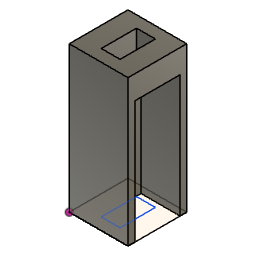
Sensor Lift (Autodesk Fusion 360 design; units mm, degrees)
Autodesk Fusion 360 part; units mm, degrees
note: some values were not read from the file. Set by a fixed rule: which sketch regions a step uses.
sketch "Sketch1" plane through (0, 0, 0) normal (0, 0, 1) x (1, 0, 0)
  line L0 (0, 0) -> (15, 0)
  line L1 (15, 0) -> (15, 15)
  line L2 (15, 15) -> (0, 15)
  line L3 (0, 15) -> (0, 0)
  line L4 (5.1406, 12.0446) -> (9.9406, 12.0446)
  line L5 (9.9406, 12.0446) -> (9.9406, 3.0446)
  line L6 (9.9406, 3.0446) -> (5.1406, 3.0446)
  line L7 (5.1406, 3.0446) -> (5.1406, 12.0446)
  dimension "d1" = 15
  dimension "d2" = 15
  dimension "d3" = 4.8
  dimension "d4" = 9
  constraint horizontal L0
  constraint vertical L1
  constraint horizontal L2
  constraint vertical L3
  constraint coincident L0.start L3.end
  constraint horizontal L4
  constraint vertical L5
  constraint horizontal L6
  constraint vertical L7
  measures "d1" distance of L0.start L2.end
  measures "d2" distance of L0.start L0.end
  measures "d3" distance of L4.start L4.end
  measures "d4" distance of L4.start L6.end
extrude "Extrude1" add sketch "Sketch1" along normal blind 37.25
sketch "Sketch4" plane through (0, 0, 0) normal (0, 0, 1) x (1, 0, 0)
  line L0 (5.0344, 1.7938) -> (15.0344, 1.7938)
  line L1 (15.0344, 1.7938) -> (15.0344, 13.2938)
  line L2 (15.0344, 13.2938) -> (5.0344, 13.2938)
  line L3 (5.0344, 13.2938) -> (5.0344, 1.7938)
  dimension "d14" = 10
  dimension "d15" = 11.5
  constraint horizontal L0
  constraint vertical L1
  constraint horizontal L2
  constraint vertical L3
  measures "d14" distance of L0.start L0.end
  measures "d15" distance of L0.start L2.end
extrude "Extrude5" cut sketch "Sketch4" along normal blind 31.25
sketch "Sketch5" plane through (15, 0, 0) normal (1, 0, 0) x (0, 1, 0)
  line L0 (13.2938, 0) -> (15, 0)
  line L1 (15, 0) -> (15, 37.25)
  line L2 (15, 37.25) -> (0, 37.25)
  line L3 (0, 37.25) -> (0, 0)
  line L4 (2.5112, 0) -> (12.5112, 0)
  line L5 (12.5112, 0) -> (12.5112, 25)
  line L6 (12.5112, 25) -> (2.5112, 25)
  line L7 (2.5112, 25) -> (2.5112, 0)
  line L8 (13.2938, 31.25) -> (13.2938, 0)
  line L9 (0, 0) -> (1.7938, 0)
  line L10 (1.7938, 0) -> (1.7938, 31.25)
  line L11 (1.7938, 31.25) -> (13.2938, 31.25)
  dimension "d18" = 25
  dimension "d21" = 10
  constraint horizontal L4
  constraint vertical L5
  constraint horizontal L6
  constraint vertical L7
  constraint coincident L0 L4.start
  measures "d18" distance of L4.start L6.end
  measures "d21" distance of L5 L7
extrude "Extrude6" cut sketch "Sketch5" against normal blind 7 contours L4 L5 L6 L7
